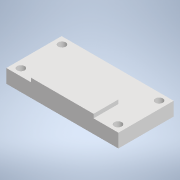
# Autodesk Inventor part: usb_camera_board
Saved by Autodesk Inventor 2022 (Build 260153000, 153)
## iProperties
Created: 2025-03-29
Part Number: usb_camera_board
Material: Типовые
Document SubType Name: Modeling
Designer: akap
Density: 1 g/cm^3
Appearance: По умолчанию
Author: akap
Autodesk Inventor part; units mm, degrees
ref_plane "YZ Plane" through (0, 0, 0) normal (1, 0, 0) x (0, 1, 0)
ref_plane "XZ Plane" through (0, 0, 0) normal (0, 1, 0) x (-1, 0, 0)
ref_plane "XY Plane" through (0, 0, 0) normal (0, 0, 1) x (1, 0, 0)
sketch "Эскиз1" plane through (0, 0, 0) normal (0, 1, 0) x (-1, 0, 0)
  line L0 (-15, 7.4) -> (15, 7.4)
  line L1 (15, 7.4) -> (15, -7.4)
  line L2 (15, -7.4) -> (-15, -7.4)
  line L3 (-15, -7.4) -> (-15, 7.4)
  line L4 (-15, 7.4) -> (15, -7.4) construction
  line L5 (15, 7.4) -> (-15, -7.4) construction
  point P0 (0, 0)
  dimension "d0" = 30
  dimension "d1" = 14.8
  constraints: 12 end point, 2 midpoint, 2 parallel, 1 horizontal, 1 perpendicular
  measures "d0" distance of L1.end L2.end
  measures "d1" distance of L0.end L1.end
extrude "Выдавливание1" add sketch "Эскиз1" along normal mid plane 3.65
sketch "Эскиз2" plane through (0, -1.825, 0) normal (0, -1, 0) x (1, 0, 0)
  line L0 (-15, 7.4) -> (15, 7.4) projected
  line L1 (8.35, 7.4) -> (-8.35, 7.4)
  line L2 (-8.35, 7.4) -> (-8.35, 0.8)
  line L3 (-8.35, 0.8) -> (8.35, 0.8)
  line L4 (8.35, 0.8) -> (8.35, 7.4)
  point P0 (0, 0)
  point P1 (0, 7.4)
  dimension "d4" = 16.7
  dimension "d5" = 6.6
  constraints: 8 end point, 2 midpoint, 2 parallel, 1 horizontal, 1 perpendicular, 1 point on line
  measures "d4" distance of L3.end L2.end
  measures "d5" distance of L2.end L1.end
extrude "Выдавливание2" add sketch "Эскиз2" against normal blind 4.7
sketch "Эскиз3" plane through (0, 1.825, 0) normal (0, 1, 0) x (1, 0, 0)
  line L0 (15, -7.4) -> (-15, -7.4) projected
  line L1 (-15, -7.4) -> (-15, 7.4) projected
  line L2 (-15, 7.4) -> (15, 7.4) projected
  line L3 (15, 7.4) -> (15, -7.4) projected
  line L4 (13, -5.5) -> (-13, -5.5)
  line L5 (-13, -5.5) -> (-13, 5.5)
  line L6 (-13, 5.5) -> (13, 5.5)
  line L7 (13, 5.5) -> (13, -5.5)
  line L8 (13, -5.5) -> (-13, 5.5) construction
  line L9 (-13, -5.5) -> (13, 5.5) construction
  circle A0 centre (-13, -5.5) radius 1
  circle A1 centre (-13, 5.5) radius 1
  circle A2 centre (13, 5.5) radius 1
  circle A3 centre (13, -5.5) radius 1
  point P0 (0, 0)
  dimension "d8" = 26
  dimension "d9" = 11
  dimension "d10" = 2
  dimension "d11" = 2
  dimension "d12" = 2
  dimension "d13" = 2
  constraints: 12 end point, 4 centre point, 4 coincident, 2 midpoint, 2 parallel, 1 horizontal, 1 perpendicular
  measures "d8" distance of L5.end L6.end
  measures "d9" distance of L4.end L5.end
  measures "d10" diameter of A0
  measures "d11" diameter of A1
  measures "d12" diameter of A2
  measures "d13" diameter of A3
extrude "Выдавливание3" cut sketch "Эскиз3" against normal blind 10 contours A0 L5 L4 | L4 L5 A0 | A3 L7 L4 | L4 L7 A3 | A1 L6 L5 | L5 L6 A1 | A2 L6 L7 | L7 L6 A2
